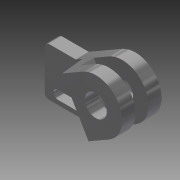
# Autodesk Inventor part: HW 7 Part 2
Saved by Autodesk Inventor 2015 (Build 190159000, 159)
## iProperties
Created: 2016-02-24
Part Number: HW 7 Part 2
Material: Steel, Carbon
Document SubType Name: Modeling
Designer: Melissa
Density: 7.85 g/cm^3
Appearance: Semi-Polished
Mass: 2270.03 g
Surface Area: 481.95 cm^2
Volume: 289.176 cm^3
Author: Melissa
Autodesk Inventor part; units mm, degrees
ref_plane "YZ Plane" through (0, 0, 0) normal (1, 0, 0) x (0, 1, 0)
ref_plane "XZ Plane" through (0, 0, 0) normal (0, 1, 0) x (-1, 0, 0)
ref_plane "XY Plane" through (0, 0, 0) normal (0, 0, 1) x (1, 0, 0)
sketch "Sketch1" plane through (0, 0, 0) normal (0, 0, 1) x (1, 0, 0)
  line L0 (6.35, 0) -> (76.2, 0)
  line L1 (76.2, 0) -> (131.1926, 31.75)
  line L2 (0, 6.35) -> (0, 63.5)
  line L3 (44.7837, 69.85) -> (93.0926, 97.7411)
  arc A0 (131.1926, 31.75) -> (93.0926, 97.7411) centre (112.1426, 64.7456) ccw
  line L4 (6.35, 69.85) -> (44.7837, 69.85)
  circle A1 centre (112.1426, 64.7456) radius 15.875
  arc A2 (6.35, 69.85) -> (0, 63.5) centre (6.35, 63.5) ccw
  arc A3 (0, 6.35) -> (6.35, 0) centre (6.35, 6.35) ccw
  line L5 (19.05, 12.7) -> (57.15, 12.7) construction
  line L6 (19.05, 6.35) -> (57.15, 6.35)
  line L7 (57.15, 19.05) -> (19.05, 19.05)
  arc A4 (19.05, 19.05) -> (19.05, 6.35) centre (19.05, 12.7) ccw
  arc A5 (57.15, 6.35) -> (57.15, 19.05) centre (57.15, 12.7) ccw
  point P0 (0, 0)
  point P1 (0, 69.85)
  point P2 (38.1, 12.7)
  dimension "d0" = 76.2
  dimension "d1" = 69.85
  dimension "d2" = 30
  dimension "d3" = 38.1
  dimension "d4" = 63.5
  dimension "d5" = 31.75
  dimension "d6" = 6.35
  dimension "d7" = 38.1
  dimension "d8" = 12.7
  dimension "d9" = 12.7
  dimension "d10" = 19.05
  constraints: 18 end point, 10 point on circle, 10 tangent, 6 centre point, 4 point on line, 3 horizontal, 2 parallel, 1 coincident, 1 equal radius, 1 midpoint, 1 vertical
  measures "d0" distance of point (0, 0) L0.end
  measures "d1" distance of point (0, 0) point (0, 69.85)
  measures "d2" angle of L0 L1
  measures "d3" radius of A0
  measures "d4" distance of L0.end L1.end
  measures "d5" diameter of A1
  measures "d6" radius of A2
  measures "d7" distance of L5.start L5.end
  measures "d8" distance between parallel lines of L6 L7
  measures "d9" distance from line of L0 point (38.1, 12.7)
  measures "d10" distance from line of L2 L5.start
extrude "Extrusion1" add sketch "Sketch1" along normal blind 19.05
sketch "Sketch2" plane through (131.1926, 31.75, 0) normal (0.5, -0.866, 0) x (0.866, 0.5, 0)
  line L0 (-63.5, 19.05) -> (0, 19.05) projected
  line L1 (0, 0) -> (-63.5, 0) projected
  line L2 (-25.4, 19.05) -> (-25.4, 57.15)
  line L3 (-25.4, 57.15) -> (-34.2411, 57.15)
  line L4 (-34.2411, 57.15) -> (-44.45, 19.05)
  point P0 (-129.4911, 0)
  dimension "d16" = 57.15
  dimension "d17" = 75
  dimension "d18" = 19.05
  dimension "d19" = 38.1
  constraints: 6 end point, 2 point on line, 1 perpendicular, 1 vertical
  measures "d16" distance from line of L1 L2.end
  measures "d17" angle of L0 L4
  measures "d18" distance of L4.end L2.start
  measures "d19" distance of L0.start L2.start
extrude "Extrusion2" add sketch "Sketch2" against normal blind 76.2
sketch "Sketch3" plane through (101.5389, 14.6294, 57.15) normal (0, 0, 1) x (0.866, 0.5, 0)
  arc A0 (34.2411, 0) -> (34.2411, 76.2) centre (34.2411, 38.1) ccw projected
  circle A1 centre (34.2411, 38.1) radius 15.875
  arc A2 (34.2411, 0) -> (34.2411, 76.2) centre (34.2411, 38.1) ccw
  line L0 (8.8411, 76.2) -> (34.2411, 76.2)
  line L1 (34.2411, 0) -> (-29.2589, 0) projected
  line L2 (8.8411, 0) -> (34.2411, 0)
  line L3 (8.8411, 76.2) -> (8.8411, 0)
  point P0 (-95.25, 38.1)
  dimension "d25" = 31.75
  dimension "d26" = 76.2
  constraints: 6 end point, 3 point on line, 2 centre point, 2 coincident, 2 point on circle, 1 horizontal, 1 perpendicular, 1 tangent
  measures "d25" diameter of A1
  measures "d26" diameter of A2
extrude "Extrusion3" add sketch "Sketch3" against normal blind 19.05
body "Solid1"
